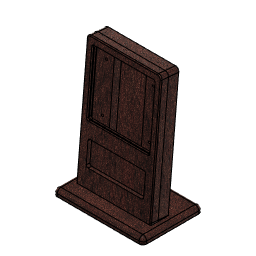
BuildStatus-Light v1 (Autodesk Fusion 360 design; units mm, degrees)
Autodesk Fusion 360 part; units mm, degrees
note: some values were not read from the file. Set by a fixed rule: which sketch regions a step uses.
sketch "Sketch1" plane through (0, 0, 0) normal (0, 1, 0) x (1, 0, 0)
  line L0 (0, 0) -> (127, 0)
  line L1 (127, 0) -> (127, -215.9)
  line L2 (127, -215.9) -> (0, -215.9)
  line L3 (0, -215.9) -> (0, 0)
  dimension "d1" = 127
  dimension "d2" = 215.9
  constraint horizontal L0
  constraint vertical L1
  constraint horizontal L2
  constraint vertical L3
  constraint coincident L0.start L3.end
  measures "d1" distance of L0.start L0.end
  measures "d2" distance of L0.start L2.end
extrude "Extrude3" add sketch "Sketch1" along normal blind 19.05 makes body 1
sketch "Sketch2" plane through (0, 19.05, 0) normal (0, 1, 0) x (-1, 0, 0)
  line L0 (0, 0) -> (0, 203.2)
  line L1 (-127, 203.2) -> (-127, 0)
  line L2 (-127, 0) -> (0, 0)
  line L3 (-6.985, 12.7) -> (-120.015, 12.7)
  line L4 (-120.015, 12.7) -> (-120.015, 139.7)
  line L5 (-120.015, 139.7) -> (-6.985, 139.7)
  line L6 (-6.985, 139.7) -> (-6.985, 12.7)
  line L7 (-14.478, 142.875) -> (-112.522, 142.875)
  line L8 (-112.522, 142.875) -> (-112.522, 202.819)
  line L9 (-112.522, 202.819) -> (-14.478, 202.819)
  line L10 (-14.478, 202.819) -> (-14.478, 142.875)
  line L11 (0, 215.9) -> (-127, 215.9)
  line L12 (-127, 215.9) -> (-127, 0)
  line L13 (-127, 0) -> (0, 0)
  line L14 (0, 0) -> (0, 215.9)
  line L15 (-36.195, 12.7) -> (-90.805, 12.7)
  line L16 (-90.805, 12.7) -> (-90.805, 139.7)
  line L17 (-90.805, 139.7) -> (-36.195, 139.7)
  line L18 (-36.195, 139.7) -> (-36.195, 12.7)
  line L19 (-22.225, 133.35) -> (-66.675, 133.35)
  line L20 (-66.675, 133.35) -> (-66.675, 152.4)
  line L21 (-66.675, 152.4) -> (-22.225, 152.4)
  line L22 (-22.225, 152.4) -> (-22.225, 133.35)
  dimension "d7" = 113.03
  dimension "d8" = 127
  dimension "d9" = 6.985
  dimension "d11" = 12.7
  dimension "d12" = 98.044
  dimension "d13" = 59.944
  dimension "d14" = 3.175
  dimension "d16" = 14.478
  dimension "d21" = 54.61
  dimension "d22" = 127
  dimension "d23" = 29.21
  dimension "d25" = 44.45
  dimension "d26" = 19.05
  dimension "d27" = 15.24
  dimension "d28" = 6.35
  constraint horizontal L3
  constraint vertical L4
  constraint horizontal L5
  constraint vertical L6
  constraint horizontal L7
  constraint vertical L8
  constraint horizontal L9
  constraint vertical L10
  constraint horizontal L15
  constraint vertical L16
  constraint horizontal L17
  constraint vertical L18
  constraint collinear L3 L15
  constraint horizontal L19
  constraint vertical L20
  constraint horizontal L21
  constraint vertical L22
  measures "d7" distance of L3.start L3.end
  measures "d8" distance of L3.start L5.end
  measures "d9" distance of L1 L4
  measures "d11" distance of L2 L3
  measures "d12" distance of L7.start L7.end
  measures "d13" distance of L7.start L9.end
  measures "d14" distance of L5 L7
  measures "d16" distance of L1 L8
  measures "d21" distance of L15.start L15.end
  measures "d22" distance of L15.start L17.end
  measures "d23" distance of L6 L18
  measures "d25" distance of L19.start L19.end
  measures "d26" distance of L19.start L21.end
  measures "d27" distance of L6 L22
  measures "d28" distance of L5 L19
extrude "Extrude4" cut sketch "Sketch2" against normal blind 12.7 contours L3 L5 L15 L16 L17 L18 L19 L20 | L5 L17 L18 L19 L20 | L5 L18 L19 L22 | L5 L7 L17 L20 L22 | L7 L20 L21 L22 bodies 1
sketch "Sketch3" plane through (0, 19.05, 0) normal (0, 1, 0) x (-1, 0, 0)
  line L0 (-66.675, 139.7) -> (-66.675, 152.4)
  line L1 (-66.675, 152.4) -> (-22.225, 152.4)
  line L2 (-22.225, 152.4) -> (-22.225, 133.35)
  line L3 (-22.225, 133.35) -> (-36.195, 133.35)
  line L4 (-36.195, 133.35) -> (-36.195, 12.7)
  line L5 (-36.195, 12.7) -> (-90.805, 12.7)
  line L6 (-90.805, 12.7) -> (-90.805, 139.7)
  line L7 (-90.805, 139.7) -> (-66.675, 139.7)
  line L8 (0, 215.9) -> (-127, 215.9)
  line L9 (-127, 215.9) -> (-127, 0)
  line L10 (-127, 0) -> (0, 0)
  line L11 (0, 0) -> (0, 215.9)
  circle A0 centre (-112.395, 134.62) radius 6.35
  line L12 (-120.015, 12.7) -> (-120.015, 139.7)
  line L13 (-120.015, 139.7) -> (-6.985, 139.7)
  circle A1 centre (-99.06, 134.62) radius 6.35
  line L14 (-127, 203.2) -> (-127, 0)
  dimension "d31" = 12.7
  dimension "d32" = 7.62
  dimension "d33" = 5.08
  dimension "d34" = 12.7
  dimension "d35" = 5.08
  dimension "d36" = 27.94
  measures "d31" diameter of A0
  measures "d32" distance of A0.centre L12
  measures "d33" distance of A0.centre L13
  measures "d34" diameter of A1
  measures "d35" distance of L13 A1.centre
  measures "d36" distance of A1.centre L14
sketch "Sketch4" plane through (0, 0, 139.7) normal (0, 0, -1) x (-1, 0, 0)
  line L0 (-66.675, 19.05) -> (-90.805, 19.05)
  line L1 (-90.805, 19.05) -> (-90.805, 6.35)
  line L2 (-90.805, 6.35) -> (-66.675, 6.35)
  line L3 (-66.675, 6.35) -> (-66.675, 19.05)
  line L4 (-90.805, 17.78) -> (-71.755, 17.78)
  line L5 (-71.755, 17.78) -> (-71.755, 6.35)
  line L6 (-71.755, 6.35) -> (-90.805, 6.35)
  line L7 (-90.805, 6.35) -> (-90.805, 17.78)
  dimension "d37" = 19.05
  dimension "d38" = 11.43
  dimension "d39" = 1.27
  constraint horizontal L4
  constraint vertical L5
  constraint horizontal L6
  constraint vertical L7
  constraint collinear L1 L7
  measures "d37" distance of L4.start L4.end
  measures "d38" distance of L4.start L1.end
  measures "d39" distance of L0 L4
extrude "Extrude5" cut sketch "Sketch4" against normal blind 6.35 contours L1 L2 L4 L5 L6 L7 bodies 1
extrude "Extrude6" cut sketch "Sketch3" against normal blind 25.4 contours A0 L13 | A0 L13 | L13 A1 | L13 A1 bodies 1
sketch "Sketch5" plane through (0, 0, 0) normal (0, -1, 0) x (1, 0, 0)
  circle A0 centre (112.395, 134.62) radius 6.35
  circle A1 centre (99.06, 134.62) radius 6.35
  line L0 (127, 215.9) -> (0, 215.9)
  line L1 (0, 215.9) -> (0, 0)
  line L2 (0, 0) -> (127, 0)
  line L3 (127, 0) -> (127, 215.9)
  line L4 (71.755, 180.975) -> (97.155, 180.975)
  line L5 (97.155, 180.975) -> (97.155, 142.875)
  line L6 (97.155, 142.875) -> (71.755, 142.875)
  line L7 (71.755, 142.875) -> (71.755, 180.975)
  dimension "d45" = 25.4
  dimension "d46" = 38.1
  dimension "d47" = 55.245
  dimension "d49" = 142.875
  constraint horizontal L4
  constraint vertical L5
  constraint horizontal L6
  constraint vertical L7
  measures "d45" distance of L4.start L4.end
  measures "d46" distance of L4.start L6.end
  measures "d47" distance of L3 L7
  measures "d49" distance of L2 L6
extrude "Extrude7" cut sketch "Sketch5" against normal blind 17.78 contours L4 L5 L6 L7 bodies 1
fillet "Fillet3" radius 3.175 4 edges at (71.755, 8.89, 180.975) (97.155, 8.89, 142.875) (71.755, 3.175, 142.875) (97.155, 8.89, 180.975) on bodies 1
fillet "Fillet4" radius 3.175 5 edges at (22.225, 12.7, 152.4) (22.225, 12.7, 133.35) (36.195, 12.7, 12.7) (90.805, 12.7, 12.7) (66.675, 12.7, 152.4) on bodies 1
fillet "Fillet5" radius 3.175 1 edges at (90.805, 18.415, 139.7) on bodies 1
fillet "Fillet6" radius 6.35 4 edges at (127, 9.525, 0) (127, 9.525, 215.9) (0, 9.525, 215.9) (0, 9.525, 0) on bodies 1
sketch "Sketch6" plane through (0, 19.05, 0) normal (0, 1, 0) x (-1, 0, 0)
  line L0 (-103.505, 110.49) -> (-23.495, 110.49)
  line L1 (-23.495, 110.49) -> (-23.495, 30.48)
  line L2 (-23.495, 30.48) -> (-103.505, 30.48)
  line L3 (-103.505, 30.48) -> (-103.505, 110.49)
  line L4 (-6.985, 12.7) -> (-120.015, 12.7)
  line L5 (-6.985, 139.7) -> (-6.985, 12.7)
  circle A0 centre (-103.505, 110.49) radius 1.75
  circle A1 centre (-23.495, 110.49) radius 1.75
  circle A2 centre (-23.495, 30.48) radius 1.75
  circle A3 centre (-103.505, 30.48) radius 1.75
  line L6 (-17.145, 145.542) -> (-109.855, 145.542)
  line L7 (-109.855, 145.542) -> (-109.855, 200.152)
  line L8 (-109.855, 200.152) -> (-17.145, 200.152)
  line L9 (-17.145, 200.152) -> (-17.145, 145.542)
  line L10 (-14.478, 142.875) -> (-112.522, 142.875)
  line L11 (-14.478, 202.819) -> (-14.478, 142.875)
  circle A4 centre (-17.145, 145.542) radius 1.75
  circle A5 centre (-109.855, 145.542) radius 1.75
  circle A6 centre (-109.855, 200.152) radius 1.75
  circle A7 centre (-17.145, 200.152) radius 1.75
  dimension "d57" = 80.01
  dimension "d58" = 80.01
  dimension "d59" = 17.78
  dimension "d60" = 16.51
  dimension "d61" = 3.5
  dimension "d62" = 3.5
  dimension "d63" = 3.5
  dimension "d64" = 3.5
  dimension "d65" = 92.71
  dimension "d66" = 54.61
  dimension "d67" = 2.667
  dimension "d68" = 2.667
  dimension "d69" = 3.5
  dimension "d70" = 3.5
  dimension "d71" = 3.5
  dimension "d72" = 3.5
  constraint horizontal L0
  constraint vertical L1
  constraint horizontal L2
  constraint vertical L3
  constraint coincident L0.start L3.end
  constraint coincident L0.end L1.start
  constraint coincident L1.end L2.start
  constraint coincident L2.end L3.start
  constraint horizontal L6
  constraint vertical L7
  constraint horizontal L8
  constraint vertical L9
  constraint coincident L6.start L9.end
  constraint coincident L6.end L7.start
  constraint coincident L7.end L8.start
  constraint coincident L8.end L9.start
  measures "d57" distance of L0.start L0.end
  measures "d58" distance of L0.start L2.end
  measures "d59" distance of L2 L4
  measures "d60" distance of L1 L5
  measures "d61" diameter of A0
  measures "d62" diameter of A1
  measures "d63" diameter of A2
  measures "d64" diameter of A3
  measures "d65" distance of L6.start L6.end
  measures "d66" distance of L6.start L8.end
  measures "d67" distance of L6 L10
  measures "d68" distance of L9 L11
  measures "d69" diameter of A4
  measures "d70" diameter of A5
  measures "d71" diameter of A6
  measures "d72" diameter of A7
extrude "Extrude8" cut sketch "Sketch6" against normal blind 12.7 contours L0 L3 A0 | L0 L3 A0 | L0 L1 A1 | L0 L1 A1 | L2 L3 A3 | L2 L3 A3 | L1 L2 A2 | L1 L2 A2 | L6 L7 A5 | L6 L7 A5 | L6 L9 A4 | L6 L9 A4 | L7 L8 A6 | L7 L8 A6 | L8 L9 A7 | L8 L9 A7 bodies 1
sketch "Sketch7" plane through (0, 0, 0) normal (0, 1, 0) x (1, 0, 0)
  line L0 (-190.5954, -4.8116) -> (-63.5954, -4.8116)
  line L1 (-63.5954, -4.8116) -> (-63.5954, -220.7116)
  line L2 (-63.5954, -220.7116) -> (-190.5954, -220.7116)
  line L3 (-190.5954, -220.7116) -> (-190.5954, -4.8116)
  dimension "d75" = 127
  dimension "d76" = 215.9
  constraint horizontal L0
  constraint vertical L1
  constraint horizontal L2
  constraint vertical L3
  measures "d75" distance of L0.start L0.end
  measures "d76" distance of L0.start L2.end
sketch "Sketch9" plane through (0, 0, 0) normal (0, 1, 0) x (1, 0, 0)
  line L0 (-181.0704, -15.6066) -> (-73.1204, -15.6066)
  line L1 (-73.1204, -15.6066) -> (-73.1204, -123.5566)
  line L2 (-73.1204, -123.5566) -> (-181.0704, -123.5566)
  line L3 (-181.0704, -123.5566) -> (-181.0704, -15.6066)
  line L4 (-190.5954, -220.7116) -> (-190.5954, -4.8116)
  line L5 (-190.5954, -4.8116) -> (-63.5954, -4.8116)
  dimension "d79" = 107.95
  dimension "d80" = 107.95
  dimension "d81" = 9.525
  dimension "d82" = 10.795
  constraint horizontal L0
  constraint vertical L1
  constraint horizontal L2
  constraint vertical L3
  measures "d79" distance of L0.start L0.end
  measures "d80" distance of L0.start L2.end
  measures "d81" distance of L3 L4
  measures "d82" distance of L0 L5
sketch "Sketch10" plane through (-127.0954, 0, 69.5816) normal (0, 1, 0) x (1, 0, 0)
  line L0 (-52.3875, 52.3875) -> (52.3875, 52.3875)
  line L1 (52.3875, 52.3875) -> (52.3875, -52.3875)
  line L2 (52.3875, -52.3875) -> (-52.3875, -52.3875)
  line L3 (-52.3875, -52.3875) -> (-52.3875, 52.3875)
  line L4 (-53.975, 53.975) -> (53.975, 53.975)
  line L5 (-53.975, -53.975) -> (-53.975, 53.975)
  dimension "d83" = 104.775
  dimension "d84" = 104.775
  dimension "d85" = 1.5875
  dimension "d86" = 1.5875
  constraint horizontal L0
  constraint vertical L1
  constraint horizontal L2
  constraint vertical L3
  measures "d83" distance of L0.start L0.end
  measures "d84" distance of L0.start L2.end
  measures "d85" distance of L0 L4
  measures "d86" distance of L3 L5
sketch "Sketch11" plane through (0, 19.05, 0) normal (0, 1, 0) x (-1, 0, 0)
sketch "Sketch12" plane through (0, 0, 0) normal (0, 1, 0) x (1, 0, 0)
  line L0 (-176.1174, -137.6536) -> (-78.0734, -137.6536)
  line L1 (-78.0734, -137.6536) -> (-78.0734, -197.5976)
  line L2 (-78.0734, -197.5976) -> (-176.1174, -197.5976)
  line L3 (-176.1174, -197.5976) -> (-176.1174, -137.6536)
  line L4 (-190.5954, -220.7116) -> (-190.5954, -4.8116)
  line L5 (-63.5954, -220.7116) -> (-190.5954, -220.7116)
  line L6 (-176.1174, -147.3056) -> (-78.0734, -147.3056)
  line L7 (-78.0734, -147.3056) -> (-78.0734, -187.9456)
  line L8 (-78.0734, -187.9456) -> (-176.1174, -187.9456)
  line L9 (-176.1174, -187.9456) -> (-176.1174, -147.3056)
  dimension "d87" = 98.044
  dimension "d88" = 59.944
  dimension "d89" = 14.478
  dimension "d90" = 23.114
  dimension "d91" = 98.044
  dimension "d92" = 40.64
  dimension "d93" = 9.652
  constraint horizontal L0
  constraint vertical L1
  constraint horizontal L2
  constraint vertical L3
  constraint horizontal L6
  constraint vertical L7
  constraint horizontal L8
  constraint vertical L9
  constraint collinear L3 L9
  measures "d87" distance of L0.start L0.end
  measures "d88" distance of L0.start L2.end
  measures "d89" distance of L3 L4
  measures "d90" distance of L2 L5
  measures "d91" distance of L6.start L6.end
  measures "d92" distance of L6.start L8.end
  measures "d93" distance of L0 L6
extrude "Extrude9" add sketch "Sketch7" against normal blind 12.7 separate body makes body 2
extrude "Extrude10" cut sketch "Sketch12" against normal blind 12.7 contours L1 L3 L6 L7 L8 L9 bodies 2
extrude "Extrude11" cut sketch "Sketch10" against normal blind 12.7 bodies 2
extrude "Extrude12" cut sketch "Sketch9" against normal blind 3.175 bodies 2
sketch "Sketch13" plane through (0, -12.7, 0) normal (0, -1, 0) x (1, 0, 0)
  line L0 (-74.7079, 121.9691) -> (-74.7079, 17.1941)
  line L1 (-74.7079, 17.1941) -> (-179.4829, 17.1941)
  line L2 (-179.4829, 17.1941) -> (-179.4829, 121.9691)
  line L3 (-179.4829, 121.9691) -> (-74.7079, 121.9691)
  line L4 (-78.0734, 187.9456) -> (-78.0734, 147.3056)
  line L5 (-78.0734, 147.3056) -> (-176.1174, 147.3056)
  line L6 (-176.1174, 147.3056) -> (-176.1174, 187.9456)
  line L7 (-176.1174, 187.9456) -> (-78.0734, 187.9456)
  line L8 (-63.5954, 220.7116) -> (-190.5954, 220.7116)
  line L9 (-190.5954, 220.7116) -> (-190.5954, 4.8116)
  line L10 (-190.5954, 4.8116) -> (-63.5954, 4.8116)
  line L11 (-63.5954, 4.8116) -> (-63.5954, 220.7116)
  line L12 (-184.2454, 17.5116) -> (-69.9454, 17.5116)
  line L13 (-69.9454, 17.5116) -> (-69.9454, 208.0116)
  line L14 (-69.9454, 208.0116) -> (-184.2454, 208.0116)
  line L15 (-184.2454, 208.0116) -> (-184.2454, 17.5116)
  dimension "d102" = 114.3
  dimension "d103" = 190.5
  dimension "d104" = 12.7
  dimension "d105" = 6.35
  constraint horizontal L12
  constraint vertical L13
  constraint horizontal L14
  constraint vertical L15
  measures "d102" distance of L12.start L12.end
  measures "d103" distance of L12.start L14.end
  measures "d104" distance of L8 L14
  measures "d105" distance of L9 L15
extrude "Extrude13" cut sketch "Sketch13" against normal blind 6.35 contours L0 L2 L3 L12 L13 L14 L15 | L0 L2 L3 L12 | L0 L1 L2 L12 | L4 L5 L6 L7 bodies 2
fillet "Fillet10" radius 6.35 4 edges at (-190.5954, -6.35, 220.7116) (-63.5954, -6.35, 220.7116) (-190.5954, -6.35, 4.8116) (-63.5954, -6.35, 4.8116) on bodies 2
sketch "Sketch14" plane through (0, 0, 0) normal (0, 1, 0) x (-1, 0, 0)
  line L0 (73.1204, 15.6066) -> (73.1204, 123.5566)
  line L1 (73.1204, 123.5566) -> (181.0704, 123.5566)
  line L2 (181.0704, 123.5566) -> (181.0704, 15.6066)
  line L3 (181.0704, 15.6066) -> (73.1204, 15.6066)
  line L4 (78.0734, 147.3056) -> (78.0734, 187.9456)
  line L5 (78.0734, 187.9456) -> (176.1174, 187.9456)
  line L6 (176.1174, 187.9456) -> (176.1174, 147.3056)
  line L7 (176.1174, 147.3056) -> (78.0734, 147.3056)
  arc A0 (63.5954, 11.1616) -> (69.9454, 4.8116) centre (69.9454, 11.1616) ccw
  line L8 (69.9454, 4.8116) -> (184.2454, 4.8116)
  arc A1 (184.2454, 4.8116) -> (190.5954, 11.1616) centre (184.2454, 11.1616) ccw
  line L9 (190.5954, 11.1616) -> (190.5954, 214.3616)
  arc A2 (190.5954, 214.3616) -> (184.2454, 220.7116) centre (184.2454, 214.3616) ccw
  line L10 (184.2454, 220.7116) -> (69.9454, 220.7116)
  arc A3 (69.9454, 220.7116) -> (63.5954, 214.3616) centre (69.9454, 214.3616) ccw
  line L11 (63.5954, 214.3616) -> (63.5954, 11.1616)
fillet "Fillet12" radius 3.175 8 edges at (-181.0704, -1.5875, 15.6066) (-179.4829, -7.9375, 17.1941) (-181.0704, -1.5875, 123.5566) (-179.4829, -4.7625, 121.9691) (-73.1204, -1.5875, 123.5566) (-74.7079, -4.7625, 121.9691) (-73.1204, -1.5875, 15.6066) (-74.7079, -7.9375, 17.1941) on bodies 2
fillet "Fillet13" radius 3.175 4 edges at (-78.0734, -3.175, 147.3056) (-176.1174, -3.175, 147.3056) (-176.1174, -3.175, 187.9456) (-78.0734, -3.175, 187.9456) on bodies 2
move_body "Move1" bodies 2 to x (1, 0, 0) y (0, 1, 0) z (0, 0, 1) at (190.5954, 31.75, -4.8116)
sketch "Sketch15" plane through (0, 0, 0) normal (0, -1, 0) x (1, 0, 0)
  circle A0 centre (99.06, 134.62) radius 6.35
  circle A1 centre (112.395, 134.62) radius 6.35
  line L0 (97.155, 177.8) -> (97.155, 146.05)
  arc A2 (93.98, 142.875) -> (97.155, 146.05) centre (93.98, 146.05) ccw
  line L1 (93.98, 142.875) -> (74.93, 142.875)
  arc A3 (71.755, 146.05) -> (74.93, 142.875) centre (74.93, 146.05) ccw
  line L2 (71.755, 146.05) -> (71.755, 177.8)
  arc A4 (74.93, 180.975) -> (71.755, 177.8) centre (74.93, 177.8) ccw
  line L3 (74.93, 180.975) -> (93.98, 180.975)
  arc A5 (97.155, 177.8) -> (93.98, 180.975) centre (93.98, 177.8) ccw
  circle A6 centre (7.9375, 207.9625) radius 4.7625
  circle A7 centre (7.9375, 207.9625) radius 1.75
  circle A8 centre (119.0625, 207.9625) radius 4.7625
  circle A9 centre (119.0625, 207.9625) radius 1.75
  circle A10 centre (7.9375, 7.9375) radius 4.7625
  circle A11 centre (7.9375, 7.9375) radius 1.75
  circle A12 centre (119.0625, 7.9375) radius 4.7625
  circle A13 centre (119.0625, 7.9375) radius 1.75
  arc A14 (0, 6.35) -> (6.35, 0) centre (6.35, 6.35) ccw
  line L4 (6.35, 0) -> (120.65, 0)
  arc A15 (120.65, 0) -> (127, 6.35) centre (120.65, 6.35) ccw
  line L5 (127, 6.35) -> (127, 209.55)
  arc A16 (127, 209.55) -> (120.65, 215.9) centre (120.65, 209.55) ccw
  line L6 (120.65, 215.9) -> (6.35, 215.9)
  arc A17 (6.35, 215.9) -> (0, 209.55) centre (6.35, 209.55) ccw
  line L7 (0, 209.55) -> (0, 6.35)
  line L8 (0, 215.9) -> (0, 0)
  line L9 (0, 0) -> (127, 0)
  line L10 (127, 0) -> (127, 215.9)
  line L11 (127, 215.9) -> (0, 215.9)
  dimension "d114" = 9.525
  dimension "d115" = 3.5
  dimension "d116" = 9.525
  dimension "d117" = 3.5
  dimension "d118" = 9.525
  dimension "d119" = 3.5
  dimension "d120" = 9.525
  dimension "d121" = 3.5
  dimension "d148" = 7.9375
  dimension "d149" = 7.9375
  dimension "d155" = 7.9375
  dimension "d156" = 7.9375
  dimension "d157" = 7.9375
  dimension "d158" = 7.9375
  dimension "d159" = 7.9375
  dimension "d160" = 7.9375
  constraint concentric A6 A7
  constraint concentric A8 A9
  constraint concentric A10 A11
  constraint concentric A12 A13
  measures "d114" diameter of A6
  measures "d115" diameter of A7
  measures "d116" diameter of A8
  measures "d117" diameter of A9
  measures "d118" diameter of A10
  measures "d119" diameter of A11
  measures "d120" diameter of A12
  measures "d121" diameter of A13
  measures "d148" distance of A10.centre L8
  measures "d149" distance of A10.centre L9
  measures "d155" distance of A12.centre L10
  measures "d156" distance of A12.centre L9
  measures "d157" distance of A8.centre L10
  measures "d158" distance of A8.centre L11
  measures "d159" distance of A6.centre L11
  measures "d160" distance of A6.centre L8
sketch "Sketch16" plane through (0, 0, 215.9) normal (0, 0, 1) x (1, 0, 0)
  line L0 (120.65, 0) -> (120.65, 19.05)
  line L1 (120.65, 19.05) -> (6.35, 19.05)
  line L2 (6.35, 19.05) -> (6.35, 0)
  circle A0 centre (31.75, 15.875) radius 6
  line L3 (6.35, 25.4) -> (120.65, 25.4)
  circle A1 centre (95.25, 15.875) radius 6
  line L4 (6.35, 0) -> (120.65, 0)
  dimension "d138" = 12
  dimension "d139" = 9.525
  dimension "d140" = 25.4
  dimension "d141" = 12
  dimension "d142" = 9.525
  dimension "d143" = 25.4
  measures "d138" diameter of A0
  measures "d139" distance of A0.centre L3
  measures "d140" distance of L2 A0.centre
  measures "d141" diameter of A1
  measures "d142" distance of L3 A1.centre
  measures "d143" distance of L0 A1.centre
extrude "Extrude22" add sketch "Sketch16" against normal blind 3 separate body contours L1 A1 | L1 A1 | L1 A0 | L1 A0 makes body 3 at (28.9218, 17.0897, 215.9) makes body 4 at (95.9807, 19.99, 212.9)
combine "Combine1" operation cut target body 1 tool bodies 4 3 keep tools
combine "Combine2" operation cut target body 2 tool bodies 4 3 keep tools
fillet "Fillet14" radius 1.5875 8 edges at (1.8599, 0, 1.8599) (63.5, 0, 0) (125.1401, 0, 1.8599) (127, 0, 107.95) (125.1401, 0, 214.0401) (63.5, 0, 215.9) (1.8599, 0, 214.0401) (0, 0, 107.95) on bodies 1
fillet "Fillet15" radius 1.5875 8 edges at (0, 31.75, 107.95) (1.8599, 31.75, 1.8599) (63.5, 31.75, 0) (125.1401, 31.75, 1.8599) (127, 31.75, 107.95) (125.1401, 31.75, 214.0401) (63.5, 31.75, 215.9) (1.8599, 31.75, 214.0401) on bodies 2
fillet "Fillet16" radius 3.175 4 edges at (120.65, 22.225, 12.7) (6.35, 22.225, 12.7) (6.35, 22.225, 203.2) (120.65, 22.225, 203.2) on bodies 2
extrude "Extrude24" cut sketch "Sketch15" against normal blind 25.4 contours A11 bodies 1 2
extrude "Extrude25" cut sketch "Sketch15" against normal blind 25.4 contours A7 bodies 1 2
extrude "Extrude26" cut sketch "Sketch15" against normal blind 25.4 contours A9 bodies 1 2
extrude "Extrude27" cut sketch "Sketch15" against normal blind 25.4 contours A13 bodies 1 2
extrude "Extrude28" cut sketch "Sketch15" against normal blind 6.35 contours A12 bodies 1
extrude "Extrude29" cut sketch "Sketch15" against normal blind 6.35 contours A10 bodies 1
extrude "Extrude30" cut sketch "Sketch15" against normal blind 6.35 contours A6 bodies 1
extrude "Extrude31" cut sketch "Sketch15" against normal blind 6.35 contours A8 bodies 1
sketch "Sketch17" plane through (0, 0, 0) normal (0, 1, 0) x (1, 0, 0)
sketch "Sketch18" plane through (0, 0, 0) normal (0, 0, 1) x (1, 0, 0)
  line L0 (-31.7871, 126.8503) -> (-184.1871, 126.8503)
  line L1 (-184.1871, 126.8503) -> (-184.1871, 25.2503)
  line L2 (-184.1871, 25.2503) -> (-31.7871, 25.2503)
  line L3 (-31.7871, 25.2503) -> (-31.7871, 126.8503)
  dimension "d175" = 152.4
  dimension "d176" = 101.6
  constraint horizontal L0
  constraint vertical L1
  constraint horizontal L2
  constraint vertical L3
  measures "d175" distance of L0.start L0.end
  measures "d176" distance of L0.start L2.end
extrude "Extrude32" add sketch "Sketch18" along normal blind 10.8857 separate body makes body 5
fillet "Fillet17" radius 6.35 4 edges at (-31.7871, 126.8503, 5.4429) (-184.1871, 126.8503, 5.4429) (-184.1871, 25.2503, 5.4429) (-31.7871, 25.2503, 5.4429) on bodies 5
fillet "Fillet18" radius 6.35 8 edges at (-107.9871, 126.8503, 0) (-182.3272, 124.9904, 0) (-184.1871, 76.0503, 0) (-182.3272, 27.1101, 0) (-107.9871, 25.2503, 0) (-33.647, 27.1101, 0) (-31.7871, 76.0503, 0) (-33.647, 124.9904, 0) on bodies 5
sketch "Sketch19" plane through (-184.1871, 0, 0) normal (-1, 0, 0) x (0, 0, 1)
  line L0 (6.35, 120.5003) -> (6.35, 31.6003)
  line L1 (6.35, 31.6003) -> (10.8857, 31.6003)
  line L2 (10.8857, 31.6003) -> (10.8857, 120.5003)
  line L3 (10.8857, 120.5003) -> (6.35, 120.5003)
  line L4 (6.35, 31.6003) -> (-3.2868, 141.7499)
  line L5 (6.35, 31.6003) -> (116.9204, 31.6003) construction
  dimension "d181" = 95
  constraint horizontal L5
  constraint coincident L0.end L1.start
  measures "d181" angle of L4 L5
ref_plane "WorkPlane1" through (-184.1871, 86.6751, 1.5316) normal (0, 0.087156, 0.996195) x (0, 0.996195, -0.087156)
sketch "Sketch20" plane through (-184.1871, 86.6751, 1.5316) normal (0, 0.087156, 0.996195) x (0, 0.996195, -0.087156)
  line L0 (14.2024, -12.7) -> (-17.5476, -12.7)
  line L1 (-17.5476, -12.7) -> (-17.5476, -139.7)
  line L2 (-17.5476, -139.7) -> (14.2024, -139.7)
  line L3 (14.2024, -139.7) -> (14.2024, -12.7)
  line L4 (33.2765, -152.4) -> (-55.2852, -152.4)
  line L5 (39.6024, -6.35) -> (39.6024, -146.05)
  dimension "d183" = 127
  dimension "d184" = 31.75
  dimension "d185" = 12.7
  dimension "d186" = 25.4
  constraint horizontal L0
  constraint vertical L1
  constraint horizontal L2
  constraint vertical L3
  measures "d183" distance of L0.start L2.end
  measures "d184" distance of L0.start L0.end
  measures "d185" distance of L2 L4
  measures "d186" distance of L3 L5
extrude "Extrude33" add sketch "Sketch20" against normal blind 25.4 separate body makes body 6
move_body "Move2" bodies 6 to x (1, 0, 0) y (0, 1, 0) z (0, 0, 1) at (0, 0.2767, 3.1629)
combine "Combine3" operation cut target body 5 tool bodies 6
sketch "Sketch21" plane through (0, 0, 133.35) normal (0, 0, 1) x (1, 0, 0)
  line L0 (25.4, 19.05) -> (25.4, 6.35)
  line L1 (25.4, 6.35) -> (36.195, 6.35)
  line L2 (36.195, 6.35) -> (36.195, 19.05)
  line L3 (36.195, 19.05) -> (25.4, 19.05)
move_body "Move3" bodies 1 2 3 4 to x (1, 0, 0) y (0, 0.996195, -0.087156) z (0, 0.087156, 0.996195) at (0, -18.5638, 3.4444)
fillet "Fillet19" radius 1.5875 4 edges at (-44.4871, 100.9489, 1.7283) (-44.4871, 69.1987, 3.1119) (-171.4871, 100.9489, 1.7283) (-171.4871, 69.1987, 3.1119) on bodies 5
fillet "Fillet20" radius 1.5875 8 edges at (-171.0221, 69.9341, 6.1833) (-107.9871, 69.4709, 6.2239) (-44.9521, 69.9341, 6.1833) (-44.4871, 85.2855, 4.8403) (-44.9521, 100.6369, 3.4972) (-107.9871, 101.1001, 3.4567) (-171.0221, 100.6369, 3.4972) (-171.4871, 85.2855, 4.8403) on bodies 5
move_body "Move4" bodies 2 1 4 3 to x (1, 0, 0) y (0, 1, 0) z (0, 0, 1) at (-166.7246, 69.2178, -212.2989)
move_body "Move5" bodies 2 4 3 1 to x (1, 0, 0) y (0, 1, 0) z (0, 0, 1) at (-5.08, 0, 0)
sketch "Sketch22" plane through (0, 1.0681, 12.2083) normal (0, -0.087156, -0.996195) x (-1, 0, 0)
  line L0 (46.0746, 70.2516) -> (169.8996, 70.2516)
  line L1 (169.8996, 70.2516) -> (169.8996, 98.8266)
  line L2 (169.8996, 98.8266) -> (46.0746, 98.8266)
  line L3 (46.0746, 98.8266) -> (46.0746, 70.2516)
  circle A0 centre (140.0546, 84.5391) radius 6
  circle A1 centre (76.5546, 84.5391) radius 6
  circle A2 centre (76.5546, 84.5391) radius 6
  circle A3 centre (140.0546, 84.5391) radius 6
  dimension "d195" = 12
  dimension "d196" = 12
  constraint concentric A1 A2
  constraint concentric A0 A3
  measures "d195" diameter of A0
  measures "d196" diameter of A1
extrude "Extrude34" add sketch "Sketch22" against normal blind 3 separate body contours A0 A3 | A1 A2 makes body 7 at (-76.1096, 80.6328, 5.2473) makes body 8 at (-135.4583, 89.3019, 6.4965)
combine "Combine4" operation cut target body 5 tool bodies 8 7 keep tools
move_body "Move6" bodies 5 1 4 3 2 7 8 to x (1, 0, 0) y (0, 0, 1) z (0, -1, 0) at (0, 120.5003, -120.5003)
equation "d16 = ( ( 5 - 3.86 ) / 2 ) * 1 in"
equation "d23 = ( ( 4.45 - 2.15 ) / 2 ) * 1 in"
equation "d67 = ( ( 2.36 - 2.15 ) / 2 ) * 1 in"
equation "d68 = ( ( 3.86 - 3.65 ) / 2 ) * 1 in"
equation "d81 = ( 0.75 / 2 ) * 1 in"
equation "d82 = ( 0.5 in + 0.175 in ) - 0.25 in"
equation "d85 = ( 1 / 16 ) * 1 in"
equation "d86 = ( 1 / 16 ) * 1 in"
equation "d93 = ( ( 2.36 - 1.6 ) / 2 ) * 1 in"
equation "d114 = ( 3 / 8 ) * 1 in"
equation "d116 = ( 3 / 8 ) * 1 in"
equation "d118 = ( 3 / 8 ) * 1 in"
equation "d120 = ( 3 / 8 ) * 1 in"
equation "d139 = ( 0.75 / 2 ) * 1 in"
equation "d142 = ( 0.75 / 2 ) * 1 in"
equation "d146 = ( 1 / 16 ) * 1 in"
equation "d147 = ( 1 / 16 ) * 1 in"
equation "d148 = ( 1 / 8 ) * 1 in + ( 0.375 / 2 ) * 1 in"
equation "d149 = ( 1 / 8 ) * 1 in + ( 0.375 / 2 ) * 1 in"
equation "d152 = ( 1 / 8 ) * 1 in"
equation "d155 = ( 1 / 8 ) * 1 in + ( 0.375 / 2 ) * 1 in"
equation "d156 = ( 1 / 8 ) * 1 in + ( 0.375 / 2 ) * 1 in"
equation "d157 = ( 1 / 8 ) * 1 in + ( 0.375 / 2 ) * 1 in"
equation "d158 = ( 1 / 8 ) * 1 in + ( 0.375 / 2 ) * 1 in"
equation "d159 = ( 1 / 8 ) * 1 in + ( 0.375 / 2 ) * 1 in"
equation "d160 = ( 1 / 8 ) * 1 in + ( 0.375 / 2 ) * 1 in"
equation "d167 = ( -1 / 4 ) * 1 in"
equation "d169 = ( -1 / 4 ) * 1 in"
equation "d171 = ( -1 / 4 ) * 1 in"
equation "d173 = ( -1 / 4 ) * 1 in"
equation "d177 = ( 3 / 7 ) * 1 in"
equation "d179 = ( 1 / 4 ) * 1 in"
equation "d180 = ( 1 / 4 ) * 1 in"
equation "d190 = ( 1 / 16 ) * 1 in"
equation "d191 = ( 1 / 16 ) * 1 in"
named bodies: "Bottom", "Top", "Left Magnet", "Right Magnet", "Stand", "Bottom Right Magnet", "Bottom Left Magnet"
